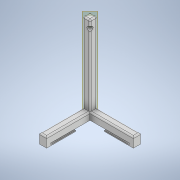
# Autodesk Inventor part: trepied
Saved by Autodesk Inventor 2022 (Build 260153000, 153)
## iProperties
Created: 2022-11-08
Part Number: trepied
Material: Generic
Document SubType Name: Modeling
Designer: 3.6b
Density: 1 g/cm^3
Appearance: Default
Author: 3.6b
Autodesk Inventor part; units mm, degrees
ref_plane "YZ Plane" through (0, 0, 0) normal (1, 0, 0) x (0, 1, 0)
ref_plane "XZ Plane" through (0, 0, 0) normal (0, 1, 0) x (-1, 0, 0)
ref_plane "XY Plane" through (0, 0, 0) normal (0, 0, 1) x (1, 0, 0)
sketch "Sketch4" plane through (0, 0, 0) normal (0, 0, 1) x (1, 0, 0)
  line L0 (0, 0) -> (25, 0)
  line L1 (25, 0) -> (25, 300)
  line L2 (25, 300) -> (0, 300)
  line L3 (0, 300) -> (0, 0)
  dimension "d16" = 25
  dimension "d17" = 300
  constraints: 8 end point, 2 parallel, 1 horizontal, 1 perpendicular
  measures "d16" distance of L2.end L1.end
  measures "d17" distance of L1.end L0.end
extrude "Extrusion4" add sketch "Sketch4" along normal blind 25
sketch "Sketch5" plane through (0, 0, 25) normal (0, 0, 1) x (1, 0, 0)
  line L0 (0, 300) -> (0, 0) projected
  line L1 (0, 0) -> (25, 0)
  line L2 (25, 0) -> (25, 25)
  line L3 (25, 25) -> (0, 25)
  line L4 (0, 25) -> (0, 0)
  dimension "d20" = 25
  dimension "d21" = 25
  constraints: 8 end point, 2 parallel, 1 horizontal, 1 perpendicular
  measures "d20" distance of L3.end L2.end
  measures "d21" distance of L2.end L1.end
extrude "Extrusion5" add sketch "Sketch5" along normal blind 150
sketch "Sketch6" plane through (25, 0, 0) normal (1, 0, 0) x (0, 0, -1)
  line L0 (0, 0) -> (0, 300) projected
  line L1 (-25, 300) -> (-25, 25) projected
  line L2 (0, 0) -> (-25, 0)
  line L3 (-25, 0) -> (-25, 25)
  line L4 (-25, 25) -> (0, 25)
  line L5 (0, 25) -> (0, 0)
  constraints: 8 end point, 2 parallel, 1 horizontal, 1 perpendicular
extrude "Extrusion6" add sketch "Sketch6" along normal blind 150
sketch "Sketch7" plane through (0, 0, 0) normal (-1, 0, 0) x (0, 0, 1)
  line L0 (0, 0) -> (175, 0) projected
  line L1 (175, 0) -> (160, 0)
  line L2 (160, 0) -> (160, -5)
  line L3 (175, -5) -> (175, 0)
  line L4 (160, -5) -> (75, -5)
  line L5 (75, -5) -> (75, -8.5)
  line L6 (75, -8.5) -> (175, -8.5)
  line L7 (175, -8.5) -> (175, -5)
  dimension "d32" = 8.5
  dimension "d33" = 85
  dimension "d34" = 100
  dimension "d37" = 3.5
  constraints: 14 end point, 3 parallel, 2 horizontal, 2 perpendicular
  measures "d32" distance of L0.end L6.end
  measures "d33" distance of L2.end L4.end
  measures "d34" distance of L5.end L6.end
  measures "d37" distance of L4.end L5.end
extrude "Extrusion7" add sketch "Sketch7" against normal blind 25
sketch "Sketch9" plane through (25, 0, 25) normal (0, 0, 1) x (1, 0, 0)
  line L0 (-25, 0) -> (150, 0) projected
  line L1 (150, 0) -> (135, 0)
  line L2 (135, 0) -> (135, -5)
  line L3 (135, -8.5) -> (150, -8.5)
  line L4 (150, -8.5) -> (150, 0)
  line L5 (135, -8.5) -> (50, -8.5)
  line L6 (50, -8.5) -> (50, -5)
  line L7 (50, -5) -> (135, -5)
  dimension "d40" = 85
  dimension "d41" = 15
  dimension "d42" = 8.5
  dimension "d43" = 3.5
  constraints: 14 end point, 3 parallel, 2 horizontal, 2 perpendicular
  measures "d40" distance of L3.start L5.end
  measures "d41" distance of L3.start L3.end
  measures "d42" distance of L3.end L0.end
  measures "d43" distance of L5.end L6.end
extrude "Extrusion8" add sketch "Sketch9" against normal blind 25
ref_plane "Work Plane2" through (0, 300, 25) normal (-0.7071068, 0, -0.7071068) x (0.7071068, 0, -0.7071068)
sketch "Sketch11" plane through (0, 300, 25) normal (-0.7071068, 0, -0.7071068) x (0.7071068, 0, -0.7071068)
  line L0 (17.6777, 275) -> (17.6777, 0) projected
  point P0 (17.6777, 300)
  point P1 (17.6777, 27.3938)
  constraints: 1 point on line
hole "Hole1" at (12.5, 272.6062, 12.5) direction (0.7071068, 0, 0.7071068) diameter 15 end through all both
fillet "Fillet6" radius 5 10 edges at (0, 132.5531, 0) (25, 162.5, 0) (0, 162.5, 25) (0, 290.0531, 0) (25, 145.0531, 25) (25, 290.0531, 25) (0, 300, 12.5) (12.5, 300, 0) (25, 300, 12.5) (12.5, 300, 25)
fillet "Fillet7" radius 5 6 edges at (0, 25, 97.5) (25, 25, 100) (12.5, 25, 175) (100, 25, 25) (97.5, 25, 0) (175, 25, 12.5)
body "Solid2"
